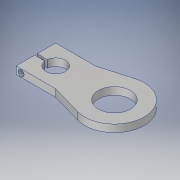
# Autodesk Inventor part: Torch Holder Base
Saved by Autodesk Inventor 2018.2 (Build 222227000, 227)
## iProperties
Created: 2018-02-18
Part Number: Torch Holder Base
Material: Aluminum 6061
Document SubType Name: Modeling
Designer: torba
Density: 2.7 g/cm^3
Appearance: Aluminum - Flat
Author: torba
Autodesk Inventor part; units mm, degrees
ref_plane "YZ Plane" through (0, 0, 0) normal (1, 0, 0) x (0, 1, 0)
ref_plane "XZ Plane" through (0, 0, 0) normal (0, 1, 0) x (-1, 0, 0)
ref_plane "XY Plane" through (0, 0, 0) normal (0, 0, 1) x (1, 0, 0)
sketch "Sketch1" plane through (0, 0, 0) normal (0, 1, 0) x (-1, 0, 0)
  circle A0 centre (0, 0) radius 12.5
  line L0 (-25.4, 25.4) -> (25.4, 25.4)
  line L1 (25.4, 25.4) -> (25.4, -25.4)
  line L2 (25.4, -25.4) -> (-25.4, -25.4)
  line L3 (-25.4, -25.4) -> (-25.4, 25.4)
  line L4 (-25.4, 25.4) -> (25.4, -25.4) construction
  line L5 (25.4, 25.4) -> (-25.4, -25.4) construction
  line L6 (-3.375, 1.5875) -> (28.375, 1.5875)
  line L7 (28.375, 1.5875) -> (28.375, -1.5875) construction
  line L8 (28.375, -1.5875) -> (-3.375, -1.5875)
  line L9 (-3.375, -1.5875) -> (-3.375, 1.5875)
  line L10 (-3.375, 1.5875) -> (28.375, -1.5875) construction
  line L11 (28.375, 1.5875) -> (-3.375, -1.5875) construction
  line L12 (25.4, 1.5875) -> (12.3988, 1.5875)
  line L13 (25.4, -1.5875) -> (12.3988, -1.5875)
  point P0 (12.5, 0)
  dimension "d0" = 25
  dimension "d2" = 50.8
  dimension "d3" = 25.4
  dimension "d4" = 25.4
  dimension "d5" = 31.75
  dimension "d6" = 3.175
  dimension "d7" = 2.975
  constraints: 28 end point, 6 point on line, 4 parallel, 3 perpendicular, 3 point on circle, 2 horizontal, 2 midpoint, 1 centre point, 1 coincident
  measures "d0" diameter of A0
  measures "d2" distance between parallel lines of L1 L3
  measures "d3" distance from line of point (0, 0) L1
  measures "d4" distance from line of point (0, 0) L0
  measures "d5" distance of L7.end L8.end
  measures "d6" distance of L6.end L7.end
  measures "d7" distance between parallel lines of L1 L7
extrude "Extrusion1" add sketch "Sketch1" along normal blind 9.525 contours A0 L8 L1 L2 L3 L0 L6
sketch "Sketch2" plane through (0, 0, 0) normal (0, -1, 0) x (1, 0, 0)
  line L0 (25.4, 25.4) -> (25.4, -25.4) projected
  line L1 (25.4, -25.4) -> (-25.4, -25.4) projected
  line L2 (-25.4, -25.4) -> (-25.4, -1.5875) projected
  line L3 (-25.4, -1.5875) -> (-12.3988, -1.5875) projected
  arc A0 (-12.3988, -1.5875) -> (-12.3988, 1.5875) centre (0, 0) ccw projected
  line L4 (-12.3988, 1.5875) -> (-25.4, 1.5875) projected
  line L5 (-25.4, 1.5875) -> (-25.4, 25.4) projected
  line L6 (-25.4, 25.4) -> (25.4, 25.4) projected
  arc A1 (-12.3988, -1.5875) -> (-12.3988, 1.5875) centre (0, 0) ccw projected
  line L7 (12.5, 0) -> (40.44, 0)
  line L8 (40.44, 0) -> (75.365, 0)
  circle A2 centre (75.365, 0) radius 20.6375
  circle A3 centre (75.365, 0) radius 38.1
  line L9 (25.4, 25.4) -> (25.4, -25.4) projected
  line L10 (25.4, 25.4) -> (64.942, 36.6466)
  line L11 (25.4, -25.4) -> (64.942, -36.6466)
  dimension "d10" = 27.94
  dimension "d11" = 34.925
  dimension "d12" = 41.275
  dimension "d13" = 76.2
  constraints: 8 end point, 4 point on circle, 2 centre point, 2 coincident, 2 horizontal, 2 tangent
  measures "d10" distance of L7.start L7.end
  measures "d11" distance of L7.end L8.end
  measures "d12" diameter of A2
  measures "d13" diameter of A3
extrude "Extrusion2" add sketch "Sketch2" against normal blind 9.525 contours L10 A3 L7 L0 | L7 A3 L11 L0 | A3
sketch "Sketch3" plane through (-25.4, 0, 25.4) normal (0, 0, 1) x (1, 0, 0)
  line L0 (0, 0) -> (50.8, 0) projected
  line L1 (50.8, 0) -> (50.8, 9.525) projected
  line L2 (0, 9.525) -> (50.8, 9.525) projected
  line L3 (0, 0) -> (0, 9.525) projected
  line L4 (0, 0) -> (13.0012, 0) projected
  line L5 (13.0012, 0) -> (13.0012, 9.525) projected
  line L6 (0, 9.525) -> (13.0012, 9.525) projected
  line L7 (0, 0) -> (0, 9.525) projected
  line L8 (0, 9.525) -> (13.0012, 0)
  line L9 (13.0012, 0) -> (13.0012, 9.525) projected
  line L10 (13.0012, 9.525) -> (0, 0)
  point P0 (25.4, 0)
  point P1 (6.5006, 4.7625)
  constraints: 4 end point, 1 midpoint
hole "Hole1" at (-18.8994, 4.7625, 25.4) direction (0, 0, -1) diameter 4.2 depth 76.2 tip angle 118 counterbore diameter 7.5 counterbore depth 6.25
body "Solid1"
